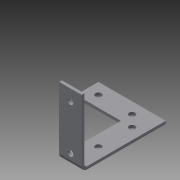
# Autodesk Inventor part: Gusset 2
Saved by Autodesk Inventor 2013 (Build 170138000, 138)
## iProperties
Created: 2013-01-31
Part Number: Gusset 2
Material: Generic
Document SubType Name: Sheet Metal
Designer: actoennies
Density: 1 g/cm^3
Sheet Metal Rule: Default
Author: actoennies
Autodesk Inventor part; units mm, degrees
ref_plane "YZ Plane" through (0, 0, 0) normal (1, 0, 0) x (0, 1, 0)
ref_plane "XZ Plane" through (0, 0, 0) normal (0, 1, 0) x (-1, 0, 0)
ref_plane "XY Plane" through (0, 0, 0) normal (0, 0, 1) x (1, 0, 0)
sketch "Sketch1" plane through (0, 0, 0) normal (0, 1, 0) x (-1, 0, 0)
  line L0 (0, 0) -> (0, 76.2)
  line L1 (25.4, 76.2) -> (25.4, 25.4)
  line L2 (25.4, 25.4) -> (76.2, 25.4)
  line L3 (76.2, 25.4) -> (76.2, 0)
  line L4 (76.2, 0) -> (0, 0)
  line L5 (25.4, 25.4) -> (0, 0) construction
  circle A0 centre (12.7, 63.5) radius 3.3782
  circle A1 centre (12.7, 25.4) radius 3.3782
  circle A2 centre (25.4, 12.7) radius 3.3782
  circle A3 centre (63.5, 12.7) radius 3.3782
  line L6 (25.4, 76.2) -> (25.4, 95.25)
  line L7 (25.4, 95.25) -> (0, 95.25)
  line L8 (0, 95.25) -> (0, 76.2)
  point P0 (0, 0)
  dimension "d0" = 76.2
  dimension "d1" = 25.4
  dimension "d2" = 50.8
  dimension "d3" = 50.8
  dimension "d4" = 25.4
  dimension "d5" = 6.7564
  dimension "d6" = 6.7564
  dimension "d7" = 6.7564
  dimension "d8" = 6.7564
  dimension "d9" = 12.7
  dimension "d10" = 0
  dimension "d11" = 12.7
  dimension "d12" = 12.7
  dimension "d13" = 12.7
  dimension "d15" = 12.7
  dimension "d17" = 19.05
  measures "d0" distance of L0.end L5.end
  measures "d1" distance of L0.end L1.start
  measures "d2" distance of L1.start L5.start
  measures "d3" distance of L5.start L2.end
  measures "d4" distance of L2.end L4.start
  measures "d5" diameter of A0
  measures "d6" diameter of A1
  measures "d7" diameter of A2
  measures "d8" diameter of A3
  measures "d9" distance from line of L4 A2.centre
  measures "d10" distance from line of L2 A1.centre
  measures "d11" distance from line of L1 A1.centre
  measures "d12" distance from line of L3 A3.centre
  measures "d13" distance from line of L4 A3.centre
  measures "d15" distance from line of L1 A0.centre
  measures "d17" distance of L1.start L6.end
extrude "Plate1" add sketch "Sketch1" along normal blind 3.175
sketch "Sketch2" plane through (0, 0, 92.075) normal (0, 0, 1) x (1, 0, 0)
  line L0 (-25.4, 0) -> (0, 0)
  line L1 (0, 0) -> (0, 76.2)
  line L2 (0, 76.2) -> (-25.4, 76.2)
  line L3 (-25.4, 76.2) -> (-25.4, 0)
  constraints: 6 end point, 1 horizontal, 1 perpendicular, 1 vertical
edge flange "Flange1" height 76.2 angle 90 thickness 3.175 bend radius 3.175 thickness toward (0, 0, 1) relief straight relief width 3.175 relief depth 1.5875 edges at (-12.7, 3.175, 95.25) wall of the first edge with corners at (-25.4, 0, 92.075) (0, 0, 92.075) (0, 76.2, 92.075) (-25.4, 76.2, 92.075)
bend "Bend1"
corner "Corner1"
sketch "Sketch3" plane through (0, 76.2, 92.075) normal (0, 0, -1) x (-1, 0, 0)
  line L0 (25.4, 0) -> (0, 0) projected
  circle A0 centre (12.7, -12.7) radius 3.3782
  circle A1 centre (12.7, -63.5) radius 3.3782
  point P0 (0, -76.2)
  dimension "d29" = 6.7564
  dimension "d30" = 6.7564
  dimension "d31" = 12.7
  dimension "d32" = 50.8
  constraints: 2 centre point
  measures "d29" diameter of A0
  measures "d30" diameter of A1
  measures "d31" distance from line of L0 A0.centre
  measures "d32" distance of A1.centre A0.centre
extrude "Cut1" cut sketch "Sketch3" against normal blind 3.175
equation "\"d33\" = Thickness"
equation "\"d19\" = BendReliefWidth"
equation "\"d20\" = BendReliefDepth"
equation "\"d21\" = MinimumRemnant"
equation "\"d22\" = BendRadius"
equation "\"d25\" = BendRadius"
equation "\"d26\" = CornerReliefSize"
equation "\"d27\" = GapSize"
equation "\"d28\" = JacobiRadiusSize"
equation "\"BendRadius\" = Thickness"
equation "\"BendReliefWidth\" = Thickness"
equation "\"BendReliefDepth\" = 0.5 * Thickness"
equation "\"CornerReliefSize\" = 4 * Thickness"
equation "\"MinimumRemnant\" = 2 * Thickness"
equation "\"TransitionRadius\" = BendRadius"
equation "\"JacobiRadiusSize\" = BendRadius"
equation "\"GapSize\" = Thickness"
equation "\"d18\" = BendRadius"
equation "\"Thickness\" = 3.175"
body "Solid1"
